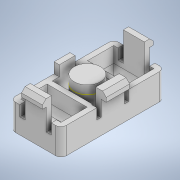
# Autodesk Inventor part: ps3buttonr1
Saved by Autodesk Inventor 2021 (Build 250183000, 183)
## iProperties
Created: 2023-05-05
Part Number: ps3buttonr1
Material: Generic
Document SubType Name: Modeling
Designer: assman
Density: 1 g/cm^3
Appearance: Default
Author: assman
## iProperties of the stored document _3DPrint.ipt
Created: 2023-05-05
Part Number: _3DPrint
Material: Generic
Document SubType Name: Modeling
Designer: assman
Density: 1 g/cm^3
Appearance: Default
Author: assman
Autodesk Inventor part; units mm, degrees
ref_plane "YZ Plane" through (0, 0, 0) normal (1, 0, 0) x (0, 1, 0)
ref_plane "XZ Plane" through (0, 0, 0) normal (0, 1, 0) x (-1, 0, 0)
ref_plane "XY Plane" through (0, 0, 0) normal (0, 0, 1) x (1, 0, 0)
sketch "Sketch1" plane through (0, 0, 0) normal (0, 1, 0) x (-1, 0, 0)
  line L0 (3.825, 9.85) -> (-3.825, 9.85)
  line L1 (-4.825, 8.85) -> (-4.825, -8.85)
  line L2 (-3.825, -9.85) -> (3.825, -9.85)
  line L3 (4.825, -8.85) -> (4.825, 8.85)
  line L4 (4.825, 9.85) -> (-4.825, -9.85) construction
  line L5 (-4.825, 9.85) -> (4.825, -9.85) construction
  arc A0 (4.825, 8.85) -> (3.825, 9.85) centre (3.825, 8.85) ccw
  arc A1 (3.825, -9.85) -> (4.825, -8.85) centre (3.825, -8.85) ccw
  arc A2 (-4.825, -8.85) -> (-3.825, -9.85) centre (-3.825, -8.85) ccw
  arc A3 (-3.825, 9.85) -> (-4.825, 8.85) centre (-3.825, 8.85) ccw
  point P0 (0, 0)
  dimension "d0" = 9.65
  dimension "d1" = 19.7
  dimension "d2" = 1
  constraints: 12 end point, 8 point on circle, 8 point on line, 8 tangent, 4 centre point, 3 equal radius, 2 midpoint, 2 parallel, 1 horizontal, 1 perpendicular
  measures "d0" distance of L5.end L4.end
  measures "d1" distance of L4.end L5.start
  measures "d2" radius of A0
extrude "Extrusion1" add sketch "Sketch1" along normal blind 5
sketch "Sketch2" plane through (0, 5, 0) normal (0, 1, 0) x (1, 0, 0)
  arc A0 (3.825, -9.85) -> (4.825, -8.85) centre (3.825, -8.85) ccw projected
  line L0 (4.825, -8.85) -> (4.825, 8.85) projected
  arc A1 (4.825, 8.85) -> (3.825, 9.85) centre (3.825, 8.85) ccw projected
  line L1 (3.825, 9.85) -> (-3.825, 9.85) projected
  arc A2 (-3.825, 9.85) -> (-4.825, 8.85) centre (-3.825, 8.85) ccw projected
  line L2 (-4.825, 8.85) -> (-4.825, -8.85) projected
  arc A3 (-4.825, -8.85) -> (-3.825, -9.85) centre (-3.825, -8.85) ccw projected
  line L3 (-3.825, -9.85) -> (3.825, -9.85) projected
  line L4 (-3.825, -8.85) -> (-3.825, 8.85)
  line L5 (-3.825, 8.85) -> (3.825, 8.85)
  line L6 (3.825, 8.85) -> (3.825, -8.85)
  line L7 (3.825, -8.85) -> (-3.825, -8.85)
  line L8 (0, -8.85) -> (0, -3.85) construction
  line L9 (0, -3.85) -> (0, -2.85) construction
  line L10 (-3.825, -2.85) -> (3.825, -2.85)
  line L11 (3.825, -2.85) -> (3.825, 2.85)
  line L12 (3.825, 2.85) -> (-3.825, 2.85)
  line L13 (-3.825, 2.85) -> (-3.825, -2.85)
  line L14 (-3.825, -2.85) -> (3.825, 2.85) construction
  line L15 (3.825, -2.85) -> (-3.825, 2.85) construction
  line L16 (-3.825, 3.85) -> (3.825, 3.85)
  line L17 (3.825, 3.85) -> (3.825, 8.85)
  line L18 (3.825, 8.85) -> (-3.825, 8.85)
  line L19 (-3.825, 8.85) -> (-3.825, 3.85)
  line L20 (-3.825, 3.85) -> (3.825, 8.85) construction
  line L21 (3.825, 3.85) -> (-3.825, 8.85) construction
  line L22 (-3.825, -8.85) -> (3.825, -8.85)
  line L23 (3.825, -8.85) -> (3.825, -3.85)
  line L24 (3.825, -3.85) -> (-3.825, -3.85)
  line L25 (-3.825, -3.85) -> (-3.825, -8.85)
  line L26 (-3.825, -8.85) -> (3.825, -3.85) construction
  line L27 (3.825, -8.85) -> (-3.825, -3.85) construction
  point P0 (0, 0)
  point P1 (0, 6.35)
  point P2 (0, -6.35)
  dimension "d5" = 1
  dimension "d6" = 5
  dimension "d8" = 1
  constraints: 48 end point, 8 midpoint, 6 parallel, 3 horizontal, 3 perpendicular, 2 point on line, 2 vertical, 3 other
  measures "d5" distance between parallel lines of L2 L4
  measures "d6" distance of L8.start L8.end
  measures "d8" distance of L8.end L9.end
extrude "Extrusion2" cut sketch "Sketch2" against normal blind 3.94 contours L4 L24 L6 L7 | L4 L12 L6 L10 | L4 L5 L6 L16
sketch "Sketch4" plane through (0, 1.06, 0) normal (0, 1, 0) x (1, 0, 0)
  line L0 (-3.825, -2.85) -> (-3.825, 2.85) construction
  line L1 (3.825, -2.85) -> (-3.825, -2.85) construction
  line L2 (3.825, 2.85) -> (3.825, -2.85) construction
  line L3 (-3.825, 2.85) -> (3.825, 2.85) construction
  circle A0 centre (0, 0) radius 2.5
  dimension "d14" = 5
  constraints: 1 centre point, 1 coincident
  measures "d14" diameter of A0
extrude "Extrusion3" add sketch "Sketch4" along normal up to surface (3.94 mm away)
sketch "Sketch5" plane through (0, 5, 0) normal (0, 1, 0) x (1, 0, 0)
  circle A0 centre (0, 0) radius 2.5 projected
thicken "Thicken1" operation add thickness 1.6 both sides no extend neighbours yes toward (0, 1, 0) faces at (1.2612, 5, 0.6619)
fillet "Fillet1" radius 1 1 edges at (-2.5, 1.06, 0)
fillet "Fillet2" radius 1 10 edges at (-3.825, 1.06, 6.35) (0, 1.06, 3.85) (0, 1.06, 8.85) (0, 1.06, -3.85) (-3.825, 1.06, -6.35) (0, 1.06, -8.85) (3.825, 1.06, -6.35) (-3.825, 1.06, 0) (3.825, 1.06, 6.35) (3.825, 1.06, 0)
sketch "Sketch6" plane through (3.825, 0, -9.85) normal (0, 0, -1) x (-1, 0, 0)
  line L0 (0, 0) -> (7.65, 0) construction
  line L1 (7.65, 0) -> (7.65, 5) construction
  line L2 (0, 5) -> (7.65, 5) construction
  line L3 (0, 0) -> (0, 5) construction
  line L4 (7.65, 5) -> (0, 5) construction
  line L5 (3.825, 5) -> (3.825, 0) construction
  line L6 (1.825, 6.75) -> (5.825, 6.75) construction
  line L7 (5.825, 6.75) -> (5.825, 3.25) construction
  line L8 (5.825, 3.25) -> (1.825, 3.25) construction
  line L9 (1.825, 3.25) -> (1.825, 6.75) construction
  line L10 (1.825, 6.75) -> (5.825, 3.25) construction
  line L11 (5.825, 6.75) -> (1.825, 3.25) construction
  line L12 (1.825, 5) -> (5.825, 5)
  line L13 (5.825, 5) -> (5.825, 8.5)
  line L14 (5.825, 8.5) -> (1.825, 8.5)
  line L15 (1.825, 8.5) -> (1.825, 5)
  dimension "d21" = 4
  dimension "d22" = 3.5
  dimension "d26" = 3.5
  constraints: 22 end point, 4 midpoint, 4 parallel, 2 horizontal, 2 perpendicular, 1 vertical
  measures "d21" distance of L7.end L8.end
  measures "d22" distance of L6.end L7.end
  measures "d26" distance of L13.end L12.end
extrude "Extrusion5" add sketch "Sketch6" against normal up to surface (1 mm away)
sketch "Sketch8" plane through (3.825, 0, -9.85) normal (0, 0, -1) x (-1, 0, 0)
  line L0 (0, 0) -> (7.65, 0) construction
  line L1 (7.65, 0) -> (7.65, 5) construction
  line L2 (5.825, 5) -> (7.65, 5) construction
  line L3 (5.825, 5) -> (5.825, 8.5) construction
  line L4 (5.825, 8.5) -> (1.825, 8.5) construction
  line L5 (1.825, 8.5) -> (1.825, 5) construction
  line L6 (0, 5) -> (1.825, 5) construction
  line L7 (0, 0) -> (0, 5) construction
  line L8 (1.825, 8.5) -> (1.825, 5) projected
  line L9 (5.825, 8.5) -> (5.825, 5) projected
  line L10 (1.825, 8.5) -> (5.825, 8.5)
  line L11 (5.825, 8.5) -> (5.825, 7.11)
  line L12 (5.825, 7.11) -> (1.825, 7.11)
  line L13 (1.825, 7.11) -> (1.825, 8.5)
  point P0 (3.825, 0)
  dimension "d29" = 1.39
  constraints: 8 end point, 2 parallel, 1 horizontal, 1 perpendicular, 1 point on line
  measures "d29" distance of L10.end L11.end
extrude "Extrusion6" add sketch "Sketch8" along normal blind 0.7
chamfer "Chamfer1" distance 0.7 angle 45 1 edges at (0, 8.5, -10.55)
sketch "Sketch9" plane through (3.825, 0, -9.85) normal (0, 0, -1) x (-1, 0, 0)
  line L0 (5.825, 7.11) -> (1.825, 7.11) construction
  line L1 (1.825, 7.11) -> (1.825, 5) construction
  line L2 (0, 5) -> (1.825, 5) construction
  line L3 (0, 0) -> (0, 5) construction
  line L4 (0, 0) -> (7.65, 0) construction
  line L5 (7.65, 0) -> (7.65, 5) construction
  line L6 (5.825, 5) -> (7.65, 5) construction
  line L7 (5.825, 5) -> (5.825, 7.11) construction
  line L8 (1.825, 5) -> (0.825, 5)
  line L9 (0.825, 5) -> (0.825, 3)
  line L10 (0.825, 3) -> (1.825, 3)
  line L11 (1.825, 3) -> (1.825, 5)
  line L12 (5.825, 5) -> (6.825, 5)
  line L13 (6.825, 5) -> (6.825, 3)
  line L14 (6.825, 3) -> (5.825, 3)
  line L15 (5.825, 3) -> (5.825, 5)
  point P0 (3.825, 0)
  dimension "d35" = 1
  dimension "d36" = 2
  dimension "d37" = 1
  dimension "d38" = 2
  constraints: 16 end point, 4 parallel, 2 horizontal, 2 perpendicular
  measures "d35" distance of L10.end L9.end
  measures "d36" distance of L9.end L8.end
  measures "d37" distance of L13.end L14.end
  measures "d38" distance of L12.end L13.end
extrude "Extrusion7" cut sketch "Sketch9" against normal up to surface (1 mm away)
mirror "Mirror1" about plane through (0, 0, 0) normal (0, 0, 1) of "Extrusion5", "Chamfer1", "Extrusion6", "Extrusion7"
sketch "Sketch10" plane through (4.825, 0, 8.85) normal (1, 0, 0) x (0, 0, -1)
  line L0 (0, 0) -> (17.7, 0) construction
  line L1 (17.7, 0) -> (17.7, 5) construction
  line L2 (0, 5) -> (17.7, 5) construction
  line L3 (0, 0) -> (0, 5) construction
  line L4 (8.85, 4.7327) -> (8.85, 0.7758) construction
  line L5 (6.625, 4.6249) -> (11.075, 4.6249) construction
  line L6 (11.075, 4.6249) -> (11.075, 2.1249) construction
  line L7 (11.075, 2.1249) -> (6.625, 2.1249) construction
  line L8 (6.625, 2.1249) -> (6.625, 4.6249) construction
  line L9 (6.625, 4.6249) -> (11.075, 2.1249) construction
  line L10 (11.075, 4.6249) -> (6.625, 2.1249) construction
  line L11 (6.625, 5) -> (11.075, 5)
  line L12 (11.075, 5) -> (11.075, 7.5)
  line L13 (11.075, 7.5) -> (6.625, 7.5)
  line L14 (6.625, 7.5) -> (6.625, 5)
  point P0 (8.85, 0)
  point P1 (8.85, 3.3749)
  dimension "d41" = 4.45
  dimension "d42" = 2.5
  dimension "d43" = 4.45
  dimension "d44" = 2.5
  constraints: 22 end point, 4 parallel, 3 point on line, 2 horizontal, 2 midpoint, 2 perpendicular, 1 vertical
  measures "d41" distance of L6.end L7.end
  measures "d42" distance of L5.end L6.end
  measures "d43" distance of L13.end L12.end
  measures "d44" distance of L12.end L11.end
extrude "Extrusion8" add sketch "Sketch10" against normal up to surface (1 mm away)
sketch "Sketch11" plane through (4.825, 0, 8.85) normal (1, 0, 0) x (0, 0, -1)
  line L0 (0, 0) -> (17.7, 0) construction
  line L1 (17.7, 0) -> (17.7, 5) construction
  line L2 (11.075, 5) -> (17.7, 5) construction
  line L3 (11.075, 5) -> (11.075, 7.5) construction
  line L4 (11.075, 7.5) -> (6.625, 7.5) construction
  line L5 (6.625, 7.5) -> (6.625, 5) construction
  line L6 (0, 5) -> (6.625, 5) construction
  line L7 (0, 0) -> (0, 5) construction
  line L8 (6.625, 5) -> (5.825, 5)
  line L9 (5.825, 5) -> (5.825, 3)
  line L10 (5.825, 3) -> (6.625, 3)
  line L11 (6.625, 3) -> (6.625, 5)
  line L12 (11.075, 5) -> (11.875, 5)
  line L13 (11.875, 5) -> (11.875, 3)
  line L14 (11.875, 3) -> (11.075, 3)
  line L15 (11.075, 3) -> (11.075, 5)
  point P0 (8.85, 0)
  dimension "d47" = 0.8
  dimension "d48" = 2
  dimension "d49" = 0.8
  dimension "d50" = 2
  constraints: 16 end point, 4 parallel, 2 horizontal, 2 perpendicular
  measures "d47" distance of L10.end L9.end
  measures "d48" distance of L9.end L8.end
  measures "d49" distance of L13.end L14.end
  measures "d50" distance of L12.end L13.end
extrude "Extrusion9" cut sketch "Sketch11" against normal up to surface (1 mm away)
sketch "Sketch12" plane through (4.825, 0, 8.85) normal (1, 0, 0) x (0, 0, -1)
  line L0 (11.875, 5) -> (11.875, 3) construction
  line L1 (11.875, 3) -> (11.075, 3) construction
  line L2 (11.075, 3) -> (11.075, 7.5) construction
  line L3 (11.075, 7.5) -> (6.625, 7.5) construction
  line L4 (6.625, 7.5) -> (6.625, 3) construction
  line L5 (6.625, 3) -> (5.825, 3) construction
  line L6 (5.825, 3) -> (5.825, 5) construction
  line L7 (0, 5) -> (5.825, 5) construction
  line L8 (0, 0) -> (0, 5) construction
  line L9 (0, 0) -> (17.7, 0) construction
  line L10 (17.7, 0) -> (17.7, 5) construction
  line L11 (11.875, 5) -> (17.7, 5) construction
  line L12 (6.625, 7.5) -> (11.075, 7.5) projected
  line L13 (11.075, 3) -> (11.075, 7.5) projected
  line L14 (6.625, 7.5) -> (11.075, 7.5)
  line L15 (11.075, 7.5) -> (11.075, 6)
  line L16 (11.075, 6) -> (6.625, 6)
  line L17 (6.625, 6) -> (6.625, 7.5)
  point P0 (8.85, 0)
  dimension "d53" = 1.5
  constraints: 8 end point, 2 parallel, 1 horizontal, 1 perpendicular, 1 point on line
  measures "d53" distance of L14.end L15.end
extrude "Extrusion10" add sketch "Sketch12" along normal blind 1
chamfer "Chamfer2" distance 0.7 angle 45 1 edges at (5.825, 7.5, 0)
sketch "Sketch13" plane through (-4.825, 0, -8.85) normal (-1, 0, 0) x (0, 0, 1)
  line L0 (0, 0) -> (17.7, 0) construction
  line L1 (17.7, 0) -> (17.7, 5) construction
  line L2 (0, 5) -> (17.7, 5) construction
  line L3 (0, 0) -> (0, 5) construction
  line L4 (0, 5) -> (17.7, 5) construction
  line L5 (8.85, 5) -> (8.85, 0) construction
  line L6 (7.35, 4.8143) -> (10.35, 4.8143) construction
  line L7 (10.35, 4.8143) -> (10.35, 2.8143) construction
  line L8 (10.35, 2.8143) -> (7.35, 2.8143) construction
  line L9 (7.35, 2.8143) -> (7.35, 4.8143) construction
  line L10 (7.35, 4.8143) -> (10.35, 2.8143) construction
  line L11 (10.35, 4.8143) -> (7.35, 2.8143) construction
  line L12 (7.35, 5) -> (10.35, 5)
  line L13 (10.35, 5) -> (10.35, 7)
  line L14 (10.35, 7) -> (7.35, 7)
  line L15 (7.35, 7) -> (7.35, 5)
  point P0 (8.85, 3.8143)
  dimension "d59" = 3
  dimension "d60" = 2
  dimension "d61" = 2
  constraints: 22 end point, 4 parallel, 3 midpoint, 3 point on line, 2 horizontal, 2 perpendicular, 1 vertical
  measures "d59" distance of L7.end L8.end
  measures "d60" distance of L6.end L7.end
  measures "d61" distance of L13.end L12.end
extrude "Extrusion11" add sketch "Sketch13" against normal up to surface (1 mm away)
sketch "Sketch14" plane through (0, 0, 0) normal (0, -1, 0) x (1, 0, 0)
  line L0 (-3.0082, -2.7578) -> (-3.0082, 2.7578) construction
  line L1 (-3.0082, 2.7578) -> (3.0082, 2.7578) construction
  line L2 (3.0082, 2.7578) -> (3.0082, -2.7578) construction
  line L3 (3.0082, -2.7578) -> (-3.0082, -2.7578) construction
  line L4 (-1.5514, -1.4223) -> (1.5514, 1.4223) construction
  line L5 (1.5514, -1.4223) -> (-1.5514, 1.4223) construction
  line L6 (-3.0082, 1.3063) -> (3.0082, 1.3063)
  line L7 (3.0082, 1.3063) -> (3.0082, -0.3557)
  line L8 (3.0082, -0.3557) -> (-0.9363, -0.3557)
  spline S0 degree 2 poles (-0.9363, -0.3557) (-0.629, -0.7599) (-0.2533, -1.5112) (-0.0768, -2.0804) knots 0 0 0 1 2 2 2
  line L9 (-0.0768, -2.0804) -> (-1.4258, -2.0804)
  spline S1 degree 2 poles (-1.4258, -2.0804) (-1.6934, -1.2437) (-2.4504, -0.3159) (-3.0082, -0.0541) knots 0 0 0 1 2 2 2
  line L10 (-3.0082, -0.0541) -> (-3.0082, 1.3063)
  point P0 (0, 0)
  point P1 (0, 0)
  point P2 (0, 0)
  constraints: 4 end point, 2 midpoint, 1 coincident, 2 other
extrude "Extrusion12" cut sketch "Sketch14" against normal blind 0.2
body "Solid1"
